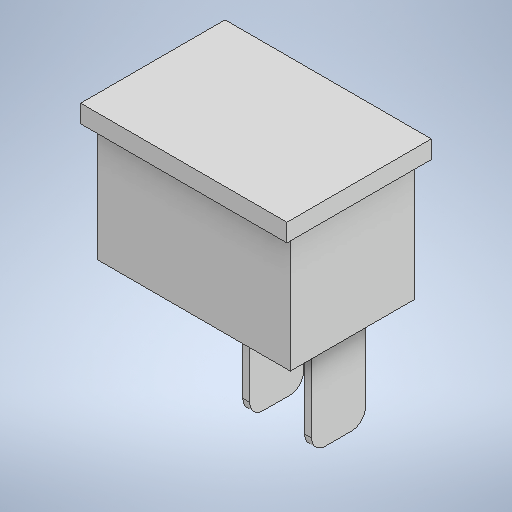
# Autodesk Inventor part: switch
Saved by Autodesk Inventor 2025.1 (Build 291241000, 241)
## iProperties
Created: 2024-09-08
Part Number: switch
Material: 一般
Document SubType Name: Modeling
Designer: right
Density: 1 g/cm^3
Appearance: 既定
Author: right
Autodesk Inventor part; units mm, degrees
ref_plane "YZ Plane" through (0, 0, 0) normal (1, 0, 0) x (0, 1, 0)
ref_plane "XZ Plane" through (0, 0, 0) normal (0, 1, 0) x (-1, 0, 0)
ref_plane "XY Plane" through (0, 0, 0) normal (0, 0, 1) x (1, 0, 0)
sketch "スケッチ1" plane through (0, 0, 0) normal (0, 1, 0) x (-1, 0, 0)
  line L0 (7, 4.5) -> (-7, 4.5)
  line L1 (-7, 4.5) -> (-7, -4.5)
  line L2 (-7, -4.5) -> (7, -4.5)
  line L3 (7, -4.5) -> (7, 4.5)
  line L4 (7, 4.5) -> (-7, -4.5) construction
  line L5 (-7, 4.5) -> (7, -4.5) construction
  point P0 (0, 0)
  dimension "d0" = 14
  dimension "d1" = 9
  constraints: 12 end point, 2 midpoint, 2 parallel, 1 horizontal, 1 perpendicular
  measures "d0" distance of L2.end L1.end
  measures "d1" distance of L1.end L0.end
extrude "押し出し1" add sketch "スケッチ1" along normal blind 8.7
sketch "スケッチ2" plane through (0, 8.7, 0) normal (0, 1, 0) x (1, 0, 0)
  line L0 (7.5, -5.25) -> (-7.5, -5.25)
  line L1 (-7.5, -5.25) -> (-7.5, 5.25)
  line L2 (-7.5, 5.25) -> (7.5, 5.25)
  line L3 (7.5, 5.25) -> (7.5, -5.25)
  line L4 (7.5, -5.25) -> (-7.5, 5.25) construction
  line L5 (-7.5, -5.25) -> (7.5, 5.25) construction
  point P0 (0, 0)
  dimension "d4" = 10.5
  dimension "d5" = 15
  constraints: 12 end point, 2 midpoint, 2 parallel, 1 horizontal, 1 perpendicular
  measures "d4" distance of L0.end L1.end
  measures "d5" distance of L0.start L0.end
extrude "押し出し2" add sketch "スケッチ2" along normal blind 1.3
sketch "スケッチ3" plane through (0, 0, 0) normal (0, -1, 0) x (1, 0, 0)
  line L0 (5.5, 1.95) -> (6, 1.95)
  line L1 (6, 1.95) -> (6, -1.95)
  line L2 (6, -1.95) -> (5.5, -1.95)
  line L3 (5.5, -1.95) -> (5.5, 1.95)
  line L4 (1, 1.95) -> (1.5, 1.95)
  line L5 (1.5, 1.95) -> (1.5, -1.95)
  line L6 (1.5, -1.95) -> (1, -1.95)
  line L7 (1, -1.95) -> (1, 1.95)
  line L8 (7, 4.5) -> (7, -4.5) projected
  point P0 (0, 0)
  point P1 (1, 0)
  point P2 (6, 0)
  point P3 (7, 0)
  dimension "d10" = 4
  dimension "d11" = 0.5
  dimension "d12" = 3.9
  dimension "d13" = 1
  constraints: 16 end point, 4 parallel, 3 midpoint, 2 horizontal, 2 perpendicular, 2 point on line, 1 collinear, 1 horizontal alignment
  measures "d10" distance between parallel lines of L5 L3
  measures "d11" distance of L5.end L6.end
  measures "d12" distance of L6.end L4.start
  measures "d13" distance of point (6, 0) point (7, 0)
extrude "押し出し3" add sketch "スケッチ3" along normal blind 7
fillet "フィレット1" radius 1 4 edges at (5.75, -7, -1.95) (5.75, -7, 1.95) (1.25, -7, -1.95) (1.25, -7, 1.95)
